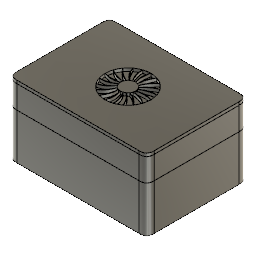
case-raspberry-pi-5-case-canakit (Autodesk Fusion 360 design; units mm, degrees)
Autodesk Fusion 360 part; units mm, degrees
sketch "Boceto1" plane through (0, 0, 0) normal (0, 0, 1) x (1, 0, 0)
  line L0 (45, 32.75) -> (-45, 32.75)
  line L1 (-45, 32.75) -> (-45, -32.75)
  line L2 (-45, -32.75) -> (45, -32.75)
  line L3 (45, -32.75) -> (45, 32.75)
  line L4 (45, 32.75) -> (-45, -32.75) construction
  line L5 (-45, 32.75) -> (45, -32.75) construction
  dimension "d1" = 65.5
  constraint horizontal L0
  constraint perpendicular L0 L1
  constraint parallel L0 L2
  constraint parallel L1 L3
  constraint coincident L4 origin
  constraint coincident L5 origin
  measures "d1" distance of L0.end L1.end
extrude "Extruir1" add sketch "Boceto1" along normal blind 30 makes body 1
fillet "Empalme1" radius 5 tangency weight 1.77315 4 edges at (-45, -32.75, 15) (-45, 32.75, 15) (45, -32.75, 15) (45, 32.75, 15) on bodies 1
shell "Vaciado1" thickness 5 removed faces 1 at (-13.3333, 10.9167, 30) on bodies 1
sketch "Boceto2" plane through (0, 0, 30) normal (0, 0, 1) x (-1, 0, 0)
  line L0 (-40, 27.75) -> (40, 27.75)
  line L1 (40, 27.75) -> (40, -27.75)
  line L2 (40, -27.75) -> (-40, -27.75)
  line L3 (-40, -27.75) -> (-40, 27.75)
  spline S0 degree 3 poles (-40, -32.75) (-41.0079, -32.75) (-41.8164, -32.6531) (-42.9382, -32.3099) (-43.3394, -32.1084) (-43.9717, -31.5941) (-44.2067, -31.3044) (-44.612, -30.5689) (-44.7613, -30.1041) (-44.9659, -28.9857) (-45, -28.3476) (-45, -27.75) knots 0 0 0 0 0.30237 0.30237 0.521848 0.521848 0.716423 0.716423 0.948779 0.948779 1.210086 1.210086 1.210086 1.210086
  line L4 (-40, -32.75) -> (40, -32.75)
  spline S1 degree 3 poles (45, -27.75) (45, -28.7579) (44.9031, -29.5664) (44.5599, -30.6882) (44.3584, -31.0894) (43.8441, -31.7217) (43.5544, -31.9567) (42.8189, -32.362) (42.3541, -32.5113) (41.2357, -32.7159) (40.5976, -32.75) (40, -32.75) knots 0 0 0 0 0.30237 0.30237 0.521848 0.521848 0.716423 0.716423 0.948779 0.948779 1.210086 1.210086 1.210086 1.210086
  line L5 (45, -27.75) -> (45, 27.75)
  spline S2 degree 3 poles (40, 32.75) (41.0079, 32.75) (41.8164, 32.6531) (42.9382, 32.3099) (43.3394, 32.1084) (43.9717, 31.5941) (44.2067, 31.3044) (44.612, 30.5689) (44.7613, 30.1041) (44.9659, 28.9857) (45, 28.3476) (45, 27.75) knots 0 0 0 0 0.30237 0.30237 0.521848 0.521848 0.716423 0.716423 0.948779 0.948779 1.210086 1.210086 1.210086 1.210086
  line L6 (40, 32.75) -> (-40, 32.75)
  spline S3 degree 3 poles (-45, 27.75) (-45, 28.7579) (-44.9031, 29.5664) (-44.5599, 30.6882) (-44.3584, 31.0894) (-43.8441, 31.7217) (-43.5544, 31.9567) (-42.8189, 32.362) (-42.3541, 32.5113) (-41.2357, 32.7159) (-40.5976, 32.75) (-40, 32.75) knots 0 0 0 0 0.30237 0.30237 0.521848 0.521848 0.716423 0.716423 0.948779 0.948779 1.210086 1.210086 1.210086 1.210086
  line L7 (-45, 27.75) -> (-45, -27.75)
  line L8 (45, 32.75) -> (-45, 32.75)
  line L9 (-45, 32.75) -> (-45, -32.75)
  line L10 (-45, -32.75) -> (45, -32.75)
  line L11 (45, -32.75) -> (45, 32.75)
  line L12 (45, 32.75) -> (-45, -32.75) construction
  line L13 (-45, 32.75) -> (45, -32.75) construction
  dimension "d7" = 90
  dimension "d8" = 65.5
  constraint horizontal L8
  constraint perpendicular L8 L9
  constraint parallel L8 L10
  constraint parallel L9 L11
  constraint coincident L12 origin
  constraint coincident L13 origin
  measures "d7" distance of L9.end L10.end
  measures "d8" distance of L8.end L9.end
extrude "Extruir1'" add sketch "Boceto2" along normal blind 15 separate body contours L0 L1 L2 L3 | S0 L9 L10 | S0 L4 S1 L5 S2 L6 S3 L7 L8 L9 L10 L11 | S1 L10 L11 | S3 L8 L9 | S2 L8 L11 makes body 2 in component "Component"
fillet "Empalme1'" radius 5 tangency weight 1.77 4 edges at (45, 32.75, 37.5) (-45, 32.75, 37.5) (-45, -32.75, 37.5) (45, -32.75, 37.5) on bodies 2 in component "Component"
shell "Vaciado1'" thickness 1 removed faces 1 at (13.3333, -10.9167, 45) on bodies 2 in component "Component"
sketch "Boceto3" plane through (0, 0, 45) normal (0, 0, 1) x (-1, 0, 0)
  spline S0 degree 3 poles (40, 31.75) (41.9289, 31.75) (42.686, 31.416) (43.1649, 30.95) (43.6556, 30.4724) (44, 29.7267) (44, 27.75) knots -1 -1 -1 -1 -0.506107 -0.506107 -0.506107 0 0 0 0
  line L0 (44, 27.75) -> (44, -27.75)
  spline S1 degree 3 poles (44, -27.75) (44, -29.6789) (43.666, -30.436) (43.2, -30.9149) (42.7224, -31.4056) (41.9767, -31.75) (40, -31.75) knots -1 -1 -1 -1 -0.506107 -0.506107 -0.506107 0 0 0 0
  line L1 (40, -31.75) -> (-40, -31.75)
  spline S2 degree 3 poles (-40, -31.75) (-41.9289, -31.75) (-42.686, -31.416) (-43.1649, -30.95) (-43.6556, -30.4724) (-44, -29.7267) (-44, -27.75) knots -1 -1 -1 -1 -0.506107 -0.506107 -0.506107 0 0 0 0
  line L2 (-44, -27.75) -> (-44, 27.75)
  spline S3 degree 3 poles (-44, 27.75) (-44, 29.6789) (-43.666, 30.436) (-43.2, 30.9149) (-42.7224, 31.4056) (-41.9767, 31.75) (-40, 31.75) knots -1 -1 -1 -1 -0.506107 -0.506107 -0.506107 0 0 0 0
  line L3 (-40, 31.75) -> (40, 31.75)
  spline S4 degree 3 poles (-45, 27.75) (-45, 28.7573) (-44.9028, 29.5657) (-44.559, 30.6878) (-44.357, 31.0891) (-43.8416, 31.722) (-43.5513, 31.9571) (-42.8106, 32.3648) (-42.3583, 32.5036) (-41.2913, 32.7129) (-40.6224, 32.75) (-40, 32.75) knots 0 0 0 0 0.302184 0.302184 0.521557 0.521557 0.716157 0.716157 0.950724 0.950724 1.270719 1.270719 1.270719 1.270719
  line L4 (-45, 27.75) -> (-45, -27.75)
  spline S5 degree 3 poles (-40, -32.75) (-41.0073, -32.75) (-41.8157, -32.6528) (-42.9378, -32.309) (-43.3391, -32.107) (-43.972, -31.5916) (-44.2071, -31.3013) (-44.6148, -30.5606) (-44.7536, -30.1083) (-44.9629, -29.0413) (-45, -28.3724) (-45, -27.75) knots 0 0 0 0 0.302184 0.302184 0.521557 0.521557 0.716157 0.716157 0.950724 0.950724 1.270719 1.270719 1.270719 1.270719
  line L5 (-40, -32.75) -> (40, -32.75)
  spline S6 degree 3 poles (45, -27.75) (45, -28.7573) (44.9028, -29.5657) (44.559, -30.6878) (44.357, -31.0891) (43.8416, -31.722) (43.5513, -31.9571) (42.8106, -32.3648) (42.3583, -32.5036) (41.2913, -32.7129) (40.6224, -32.75) (40, -32.75) knots 0 0 0 0 0.302184 0.302184 0.521557 0.521557 0.716157 0.716157 0.950724 0.950724 1.270719 1.270719 1.270719 1.270719
  line L6 (45, -27.75) -> (45, 27.75)
  spline S7 degree 3 poles (40, 32.75) (41.0073, 32.75) (41.8157, 32.6528) (42.9378, 32.309) (43.3391, 32.107) (43.972, 31.5916) (44.2071, 31.3013) (44.6148, 30.5606) (44.7536, 30.1083) (44.9629, 29.0413) (45, 28.3724) (45, 27.75) knots 0 0 0 0 0.302184 0.302184 0.521557 0.521557 0.716157 0.716157 0.950724 0.950724 1.270719 1.270719 1.270719 1.270719
  line L7 (40, 32.75) -> (-40, 32.75)
  line L8 (33.5871, 31.75) -> (28.5871, 31.75)
  line L9 (28.5871, 31.75) -> (28.5871, -31.75)
  line L10 (28.5871, -31.75) -> (33.5871, -31.75)
  line L11 (33.5871, -31.75) -> (33.5871, 31.75)
  dimension "d14" = 5
  constraint horizontal L8
  constraint vertical L9
  constraint horizontal L10
  constraint vertical L11
  constraint coincident L3 L8.start
  measures "d14" distance of L8.start L8.end
extrude "Extruir2" add sketch "Boceto3" along normal blind 0.5 separate body contours L1 L3 L8 L9 L10 L11 makes body 3
move_body "Desplazar1" bodies 3 to x (1, 0, 0) y (0, 1, 0) z (0, 0, 1) at (0, 0, -0.5)
sketch "Boceto4" plane through (0, 0, 45) normal (0, 0, 1) x (-1, 0, 0)
  spline S0 degree 3 poles (40, 31.75) (41.9289, 31.75) (42.686, 31.416) (43.1649, 30.95) (43.6556, 30.4724) (44, 29.7267) (44, 27.75) knots -1 -1 -1 -1 -0.506107 -0.506107 -0.506107 0 0 0 0
  line L0 (44, 27.75) -> (44, -27.75)
  spline S1 degree 3 poles (44, -27.75) (44, -29.6789) (43.666, -30.436) (43.2, -30.9149) (42.7224, -31.4056) (41.9767, -31.75) (40, -31.75) knots -1 -1 -1 -1 -0.506107 -0.506107 -0.506107 0 0 0 0
  line L1 (40, -31.75) -> (-40, -31.75)
  spline S2 degree 3 poles (-40, -31.75) (-41.9289, -31.75) (-42.686, -31.416) (-43.1649, -30.95) (-43.6556, -30.4724) (-44, -29.7267) (-44, -27.75) knots -1 -1 -1 -1 -0.506107 -0.506107 -0.506107 0 0 0 0
  line L2 (-44, -27.75) -> (-44, 27.75)
  spline S3 degree 3 poles (-44, 27.75) (-44, 29.6789) (-43.666, 30.436) (-43.2, 30.9149) (-42.7224, 31.4056) (-41.9767, 31.75) (-40, 31.75) knots -1 -1 -1 -1 -0.506107 -0.506107 -0.506107 0 0 0 0
  line L3 (-40, 31.75) -> (40, 31.75)
  spline S4 degree 3 poles (-45, 27.75) (-45, 28.7573) (-44.9028, 29.5657) (-44.559, 30.6878) (-44.357, 31.0891) (-43.8416, 31.722) (-43.5513, 31.9571) (-42.8106, 32.3648) (-42.3583, 32.5036) (-41.2913, 32.7129) (-40.6224, 32.75) (-40, 32.75) knots 0 0 0 0 0.302184 0.302184 0.521557 0.521557 0.716157 0.716157 0.950724 0.950724 1.270719 1.270719 1.270719 1.270719
  line L4 (-45, 27.75) -> (-45, -27.75)
  spline S5 degree 3 poles (-40, -32.75) (-41.0073, -32.75) (-41.8157, -32.6528) (-42.9378, -32.309) (-43.3391, -32.107) (-43.972, -31.5916) (-44.2071, -31.3013) (-44.6148, -30.5606) (-44.7536, -30.1083) (-44.9629, -29.0413) (-45, -28.3724) (-45, -27.75) knots 0 0 0 0 0.302184 0.302184 0.521557 0.521557 0.716157 0.716157 0.950724 0.950724 1.270719 1.270719 1.270719 1.270719
  line L5 (-40, -32.75) -> (40, -32.75)
  spline S6 degree 3 poles (45, -27.75) (45, -28.7573) (44.9028, -29.5657) (44.559, -30.6878) (44.357, -31.0891) (43.8416, -31.722) (43.5513, -31.9571) (42.8106, -32.3648) (42.3583, -32.5036) (41.2913, -32.7129) (40.6224, -32.75) (40, -32.75) knots 0 0 0 0 0.302184 0.302184 0.521557 0.521557 0.716157 0.716157 0.950724 0.950724 1.270719 1.270719 1.270719 1.270719
  line L6 (45, -27.75) -> (45, 27.75)
  spline S7 degree 3 poles (40, 32.75) (41.0073, 32.75) (41.8157, 32.6528) (42.9378, 32.309) (43.3391, 32.107) (43.972, 31.5916) (44.2071, 31.3013) (44.6148, 30.5606) (44.7536, 30.1083) (44.9629, 29.0413) (45, 28.3724) (45, 27.75) knots 0 0 0 0 0.302184 0.302184 0.521557 0.521557 0.716157 0.716157 0.950724 0.950724 1.270719 1.270719 1.270719 1.270719
  line L7 (40, 32.75) -> (-40, 32.75)
  line L8 (45, 32.75) -> (-45, 32.75)
  line L9 (-45, 32.75) -> (-45, -32.75)
  line L10 (-45, -32.75) -> (45, -32.75)
  line L11 (45, -32.75) -> (45, 32.75)
  line L12 (45, 32.75) -> (-45, -32.75) construction
  line L13 (-45, 32.75) -> (45, -32.75) construction
  dimension "d17" = 90
  dimension "d18" = 65.5
  constraint horizontal L8
  constraint perpendicular L8 L9
  constraint parallel L8 L10
  constraint parallel L9 L11
  constraint coincident L12 origin
  constraint coincident L13 origin
  measures "d17" distance of L9.end L10.end
  measures "d18" distance of L8.end L9.end
extrude "Extruir1''" add sketch "Boceto4" along normal blind 2 separate body contours S0 L0 S1 L1 S2 L2 S3 L3 | S4 L8 L9 | S4 L4 S5 L5 S6 L6 S7 L7 L8 L9 L10 L11 | S5 L9 L10 | S7 L8 L11 | S6 L10 L11 makes body 4 in component "Component'"
fillet "Empalme1''" radius 5 tangency weight 1.77 4 edges at (45, 32.75, 46) (-45, 32.75, 46) (-45, -32.75, 46) (45, -32.75, 46) on bodies 4 in component "Component'"
hole "Agujero1" at (0, 0, 47) direction (0, 0, -1) diameter 30 depth 2 tip angle 180 bodies 4 in component "Component'"
sketch "Boceto5" plane through (0, 0, 47) normal (0, 0, 1) x (-1, 0, 0)
  circle A0 centre (0, 0) radius 15
  spline S0 degree 3 poles (-45, 27.75) (-45, 28.7573) (-44.9028, 29.5657) (-44.559, 30.6878) (-44.357, 31.0891) (-43.8416, 31.722) (-43.5513, 31.9571) (-42.8106, 32.3648) (-42.3583, 32.5036) (-41.2913, 32.7129) (-40.6224, 32.75) (-40, 32.75) knots 0 0 0 0 0.302184 0.302184 0.521557 0.521557 0.716157 0.716157 0.950724 0.950724 1.270719 1.270719 1.270719 1.270719
  line L0 (-45, 27.75) -> (-45, -27.75)
  spline S1 degree 3 poles (-40, -32.75) (-41.0073, -32.75) (-41.8157, -32.6528) (-42.9378, -32.309) (-43.3391, -32.107) (-43.972, -31.5916) (-44.2071, -31.3013) (-44.6148, -30.5606) (-44.7536, -30.1083) (-44.9629, -29.0413) (-45, -28.3724) (-45, -27.75) knots 0 0 0 0 0.302184 0.302184 0.521557 0.521557 0.716157 0.716157 0.950724 0.950724 1.270719 1.270719 1.270719 1.270719
  line L1 (-40, -32.75) -> (40, -32.75)
  spline S2 degree 3 poles (45, -27.75) (45, -28.7573) (44.9028, -29.5657) (44.559, -30.6878) (44.357, -31.0891) (43.8416, -31.722) (43.5513, -31.9571) (42.8106, -32.3648) (42.3583, -32.5036) (41.2913, -32.7129) (40.6224, -32.75) (40, -32.75) knots 0 0 0 0 0.302184 0.302184 0.521557 0.521557 0.716157 0.716157 0.950724 0.950724 1.270719 1.270719 1.270719 1.270719
  line L2 (45, -27.75) -> (45, 27.75)
  spline S3 degree 3 poles (40, 32.75) (41.0073, 32.75) (41.8157, 32.6528) (42.9378, 32.309) (43.3391, 32.107) (43.972, 31.5916) (44.2071, 31.3013) (44.6148, 30.5606) (44.7536, 30.1083) (44.9629, 29.0413) (45, 28.3724) (45, 27.75) knots 0 0 0 0 0.302184 0.302184 0.521557 0.521557 0.716157 0.716157 0.950724 0.950724 1.270719 1.270719 1.270719 1.270719
  line L3 (40, 32.75) -> (-40, 32.75)
  circle A1 centre (0, 0) radius 5
  dimension "d26" = 10
  constraint coincident A0.centre A1.centre
  measures "d26" diameter of A1
extrude "Extruir3" add sketch "Boceto5" along normal blind 2 separate body contours A1 makes body 5
move_body "Desplazar2" bodies 5 to x (1, 0, 0) y (0, 1, 0) z (0, 0, 1) at (0, 0, -2)
sketch "Boceto6" plane through (0, 0, 45) normal (0, 0, -1) x (1, 0, 0)
  circle A0 centre (0, 0) radius 5
  arc A1 (-5, 0) -> (-15, 0) centre (-10, -20.4785) ccw
  line L0 (5, 0) -> (-5, 0)
  line L1 (0, 5) -> (0, -5)
  arc A2 (-5, 0) -> (-15, 0) centre (-10, -11.5) ccw
  arc A3 (-4.7553, -1.5451) -> (-14.2658, -4.6353) centre (-5.9569, -14.0273) ccw
  arc A4 (-4.7553, -1.5451) -> (-14.2658, -4.6353) centre (-3.1824, -22.5663) ccw
  arc A5 (-4.0451, -2.9389) -> (-12.1353, -8.8168) centre (-1.3306, -15.1815) ccw
  arc A6 (-4.0451, -2.9389) -> (-12.1353, -8.8168) centre (3.9468, -22.4453) ccw
  arc A7 (-2.9389, -4.0451) -> (-8.8168, -12.1353) centre (3.4258, -14.8497) ccw
  arc A8 (-2.9389, -4.0451) -> (-8.8168, -12.1353) centre (10.6896, -20.1271) ccw
  arc A9 (-1.5451, -4.7553) -> (-4.6353, -14.2658) centre (7.847, -13.0643) ccw
  arc A10 (-1.5451, -4.7553) -> (-4.6353, -14.2658) centre (16.386, -15.8388) ccw
  arc A11 (0, -5) -> (0, -15) centre (11.5, -10) ccw
  arc A12 (0, -5) -> (0, -15) centre (20.4785, -10) ccw
  arc A13 (1.5451, -4.7553) -> (4.6353, -14.2658) centre (14.0273, -5.9569) ccw
  arc A14 (1.5451, -4.7553) -> (4.6353, -14.2658) centre (22.5663, -3.1824) ccw
  arc A15 (2.9389, -4.0451) -> (8.8168, -12.1353) centre (15.1815, -1.3306) ccw
  arc A16 (2.9389, -4.0451) -> (8.8168, -12.1353) centre (22.4453, 3.9468) ccw
  arc A17 (4.0451, -2.9389) -> (12.1353, -8.8168) centre (14.8497, 3.4258) ccw
  arc A18 (4.0451, -2.9389) -> (12.1353, -8.8168) centre (20.1271, 10.6896) ccw
  arc A19 (4.7553, -1.5451) -> (14.2658, -4.6353) centre (13.0643, 7.847) ccw
  arc A20 (4.7553, -1.5451) -> (14.2658, -4.6353) centre (15.8388, 16.386) ccw
  arc A21 (5, 0) -> (15, 0) centre (10, 11.5) ccw
  arc A22 (5, 0) -> (15, 0) centre (10, 20.4785) ccw
  arc A23 (4.7553, 1.5451) -> (14.2658, 4.6353) centre (5.9569, 14.0273) ccw
  arc A24 (4.7553, 1.5451) -> (14.2658, 4.6353) centre (3.1824, 22.5663) ccw
  arc A25 (4.0451, 2.9389) -> (12.1353, 8.8168) centre (1.3306, 15.1815) ccw
  arc A26 (4.0451, 2.9389) -> (12.1353, 8.8168) centre (-3.9468, 22.4453) ccw
  arc A27 (2.9389, 4.0451) -> (8.8168, 12.1353) centre (-3.4258, 14.8497) ccw
  arc A28 (2.9389, 4.0451) -> (8.8168, 12.1353) centre (-10.6896, 20.1271) ccw
  arc A29 (1.5451, 4.7553) -> (4.6353, 14.2658) centre (-7.847, 13.0643) ccw
  arc A30 (1.5451, 4.7553) -> (4.6353, 14.2658) centre (-16.386, 15.8388) ccw
  arc A31 (0, 5) -> (0, 15) centre (-11.5, 10) ccw
  arc A32 (0, 5) -> (0, 15) centre (-20.4785, 10) ccw
  arc A33 (-1.5451, 4.7553) -> (-4.6353, 14.2658) centre (-14.0273, 5.9569) ccw
  arc A34 (-1.5451, 4.7553) -> (-4.6353, 14.2658) centre (-22.5663, 3.1824) ccw
  arc A35 (-2.9389, 4.0451) -> (-8.8168, 12.1353) centre (-15.1815, 1.3306) ccw
  arc A36 (-2.9389, 4.0451) -> (-8.8168, 12.1353) centre (-22.4453, -3.9468) ccw
  arc A37 (-4.0451, 2.9389) -> (-12.1353, 8.8168) centre (-14.8497, -3.4258) ccw
  arc A38 (-4.0451, 2.9389) -> (-12.1353, 8.8168) centre (-20.1271, -10.6896) ccw
  arc A39 (-4.7553, 1.5451) -> (-14.2658, 4.6353) centre (-13.0643, -7.847) ccw
  arc A40 (-4.7553, 1.5451) -> (-14.2658, 4.6353) centre (-15.8388, -16.386) ccw
  dimension "d30" = 360
  constraint coincident A0 A1.start
  constraint coincident A0 L0.start
  constraint horizontal L0
  constraint coincident A0 L1.start
  constraint coincident A0 L1.end
  constraint perpendicular L0 L1
extrude "Extruir4" add sketch "Boceto6" against normal blind 2 separate body contours A19 A20 | A17 A18 | A15 A16 | A13 A14 | A11 A12 | A9 A10 | A7 A8 | A5 A6 | A3 A4 | A1 A2 | A39 A40 | A37 A38 | A35 A36 | A33 A34 | A31 A32 | A29 A30 | A27 A28 | A25 A26 | A23 A24 | A21 A22 makes body 6 at (-8.3312, -11.8341, 46.3333) makes body 7 at (3.4245, -4.3462, 45.6667) makes body 8 at (10.2907, 4.3824, 46.3333) makes body 9 at (-1.0269, 9.4288, 46.3333) makes body 10 at (-13.8294, 4.2665, 46.3333) makes body 11 at (-9.5942, 5.7495, 46.3333) makes body 12 at (3.2847, 12.4257, 46.3333) makes body 13 at (5.5291, 0.2158, 45.6667) makes body 14 at (4.6463, -11.9833, 46.3333) makes body 15 at (-7.0244, -6.3729, 46.3333) makes body 16 at (-1.5033, -5.3251, 45.6667) makes body 17 at (9.5942, -5.7495, 46.3333) makes body 18 at (8.4328, 7.3479, 46.3333) makes body 19 at (-4.677, 13.696, 46.3333) makes body 20 at (-7.7269, -0.8322, 46.3333) makes body 21 at (-8.6804, 11.5804, 46.3333) makes body 22 at (3.0753, 4.6, 45.6667) makes body 23 at (7.6059, -1.5963, 46.3333) makes body 24 at (0.8322, -7.7269, 46.3333) makes body 25 at (-7.0915, -3.1792, 46.3333)
component "Component" placed x (1, 0, 0) y (0, 1, 0) z (0, 0, 1) at (0, 0, 0)
component "Component'" placed x (1, 0, 0) y (0, 1, 0) z (0, 0, 1) at (0, 0, 0)
